shankTop.5in_v14 (Autodesk Fusion 360 design; units mm, degrees)
Autodesk Fusion 360 part; units mm, degrees
sketch "Sketch1" plane through (0, 0, 0) normal (0, 0, 1) x (1, 0, 0)
  line L0 (10.9985, -6.35) -> (0, 12.7)
  line L1 (0, 12.7) -> (-10.9985, -6.35)
  line L2 (-10.9985, -6.35) -> (10.9985, -6.35)
  line L3 (3.6662, -6.35) -> (7.3323, 0) construction
  line L4 (7.3323, 0) -> (3.6662, 6.35) construction
  line L5 (3.6662, 6.35) -> (-3.6662, 6.35) construction
  line L6 (-3.6662, 6.35) -> (-7.3323, 0) construction
  line L7 (-7.3323, 0) -> (-3.6662, -6.35) construction
  line L8 (-3.6662, -6.35) -> (3.6662, -6.35) construction
  circle A0 centre (0, 0) radius 12.7
  arc A1 (3.2996, 6.985) -> (-3.2996, 6.985) centre (0, 5.08) ccw
  arc A2 (-7.699, -0.635) -> (-4.3994, -6.35) centre (-4.3994, -2.54) ccw
  arc A3 (4.3994, -6.35) -> (7.699, -0.635) centre (4.3994, -2.54) ccw
  dimension "d1" = 6.35
  dimension "d2" = 25.4
  dimension "d4" = 3.81
  dimension "d6" = 360
  constraint coincident A0.centre origin
  constraint horizontal L2
  constraint collinear L2 L8
  constraint coincident L0 A1.start
  constraint coincident L1 A1.end
  constraint horizontal A1.start A1.end
  constraint tangent L0 A1
  measures "d1" distance of A0.centre L2
  measures "d2" diameter of A0
  measures "d4" radius of A1
extrude "Extrude1" add sketch "Sketch1" along normal blind 12.7 contours L0 L2 A3 | L2 A0 | L0 A0 | L1 A0 | L1 L2 A2 | L0 L1 A1
sketch "Sketch2" plane through (0, 0, 0) normal (0, 1, 0) x (1, 0, 0)
  line L0 (0, -12.7) -> (0, -15.875)
  line L1 (-12.7, -12.7) -> (12.7, -12.7)
  line L2 (-12.7, 0) -> (12.7, 0)
  line L3 (12.7, -12.7) -> (12.7, -15.875)
  line L4 (0, -15.875) -> (12.7, -15.875)
  line L5 (0, 0) -> (0, -3.175) construction
  line L6 (0, -3.175) -> (0, -6.35) construction
  line L7 (0, -6.35) -> (0, -9.525) construction
  line L8 (0, -9.525) -> (0, -12.7) construction
  point P0 (0, -9.525)
  point P1 (0, -6.35)
  point P2 (0, -3.175)
  dimension "d9" = 3.175
  dimension "d10" = 12.7
  constraint vertical L0
  constraint coincident L1.end L3.start
  constraint perpendicular L0 L4
  constraint coincident L0.start L1
  constraint vertical L5.start L0.start
  constraint coincident L5.start origin
  constraint perpendicular L2 L5
  constraint perpendicular L2 L6
  constraint perpendicular L2 L7
  constraint perpendicular L1 L8
  constraint coincident P0 L7.end
  constraint coincident P1 L6.end
  constraint coincident P2 L5.end
  constraint equal L7 L8
  constraint equal L6 L7
  constraint equal L5 L6
  measures "d9" distance of L0.start L0.end
  measures "d10" distance of L0.end L3.end
revolve "Revolve1" add sketch "Sketch2" angle 360 about axis through (0, 0, 12.7) along (0, 0, 1)
sketch "Sketch3" plane through (0, 0, 15.875) normal (0, 0, 1) x (-1, 0, 0)
  circle A0 centre (0, 0) radius 12.7
  circle A1 centre (0, 0) radius 6.35
  dimension "d12" = 12.7
  constraint coincident A0.centre A1.centre
  measures "d12" diameter of A1
extrude "Extrude2" add sketch "Sketch3" along normal blind 25.4 contours A1
sketch "Sketch4" plane through (0, 0, 0) normal (1, 0, 0) x (0, 1, 0)
  line L0 (6.35, 41.275) -> (-6.35, 41.275)
  line L1 (-6.35, 15.875) -> (-6.35, 24.765) construction
  line L2 (-6.35, 24.765) -> (-4.826, 27.4046)
  line L3 (-4.826, 27.4046) -> (-4.826, 35.7866)
  line L4 (-4.826, 35.7866) -> (-6.35, 38.4263)
  line L5 (-6.35, 41.275) -> (-6.35, 38.4263) construction
  line L6 (-6.35, 38.4263) -> (-6.35, 24.765)
  line L7 (-6.35, 15.875) -> (6.35, 15.875)
  dimension "d15" = 8.89
  dimension "d16" = 8.382
  dimension "d17" = 150
  dimension "d18" = 150
  dimension "d19" = 1.524
  constraint vertical L3
  constraint vertical L0.end L4.end
  constraint coincident L0.end L5.start
  measures "d15" distance of L1.start L1.end
  measures "d16" distance of L2.end L3.end
  measures "d17" angle of L2 L3
  measures "d18" angle of L3 L4
  measures "d19" distance of L1 L3
extrude "Extrude3" cut sketch "Sketch4" along normal mid plane 12.7
hole "Hole1" at (0, 0, 9.525) at (0, 0, 3.175) direction (0, -1, 0) diameter 2.7686 depth 12.7 tip angle 180
thread "Thread1" "ANSI Unified Screw Threads 0.138(#6) 6-32 UNC 3B"
pattern_circular "C-Pattern1" count 3 over 360 about axis through (0, 0, 0) along (0, 0, 1) of "Hole1"
equation "d7 = shankLength"
equation "d18 = d17"
equation "d20 = d12 / 2"
equation "shankLength = 0.5 in"
